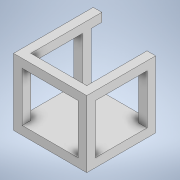
# Autodesk Inventor part: Pump and motor housing new
Saved by Autodesk Inventor 2021 (Build 250183000, 183)
## iProperties
Created: 2020-10-21
Part Number: Pump and motor housing new
Material: Generic
Document SubType Name: Modeling
Designer: nabee
Density: 1 g/cm^3
Appearance: Default
Author: nabee
Autodesk Inventor part; units mm, degrees
ref_plane "YZ Plane" through (0, 0, 0) normal (1, 0, 0) x (0, 1, 0)
ref_plane "XZ Plane" through (0, 0, 0) normal (0, 1, 0) x (-1, 0, 0)
ref_plane "XY Plane" through (0, 0, 0) normal (0, 0, 1) x (1, 0, 0)
sketch "Sketch1" plane through (0, 0, 0) normal (0, 0, 1) x (1, 0, 0)
  line L0 (0, 0) -> (170, 0)
  line L1 (170, 0) -> (170, 310)
  line L2 (170, 310) -> (0, 310)
  line L3 (0, 310) -> (0, 0)
  dimension "d0" = 310
  dimension "d1" = 170
  constraints: 8 end point, 2 parallel, 1 horizontal, 1 perpendicular
  measures "d0" distance of L2.end L0.start
  measures "d1" distance of L0.start L0.end
extrude "Extrusion1" add sketch "Sketch1" along normal blind 150
sketch "Sketch2" plane through (0, 0, 150) normal (0, 0, 1) x (1, 0, 0)
  line L0 (20, 290) -> (150, 290)
  line L1 (150, 290) -> (150, 20)
  line L2 (150, 20) -> (20, 20)
  line L3 (20, 20) -> (20, 290)
  line L4 (170, 310) -> (0, 310) projected
  line L5 (0, 310) -> (0, 0) projected
  line L6 (0, 0) -> (170, 0) projected
  line L7 (170, 0) -> (170, 310) projected
  dimension "d4" = 20
  dimension "d5" = 20
  dimension "d6" = 20
  dimension "d7" = 20
  constraints: 8 end point, 2 parallel, 1 horizontal, 1 perpendicular
  measures "d4" distance between parallel lines of L4 L0
  measures "d5" distance between parallel lines of L5 L3
  measures "d6" distance between parallel lines of L6 L2
  measures "d7" distance between parallel lines of L7 L1
sketch "Sketch3" plane through (0, 310, 0) normal (0, 1, 0) x (1, 0, 0)
  line L0 (20, -20) -> (150, -20)
  line L1 (150, -20) -> (150, -130)
  line L2 (150, -130) -> (20, -130)
  line L3 (20, -130) -> (20, -20)
  line L4 (170, 0) -> (0, 0) projected
  line L5 (0, 0) -> (0, -150) projected
  line L6 (170, -150) -> (0, -150) projected
  line L7 (170, 0) -> (170, -150) projected
  dimension "d8" = 20
  dimension "d9" = 20
  dimension "d10" = 20
  dimension "d11" = 20
  constraints: 8 end point, 2 parallel, 1 horizontal, 1 perpendicular
  measures "d8" distance between parallel lines of L4 L0
  measures "d9" distance between parallel lines of L5 L3
  measures "d10" distance between parallel lines of L6 L2
  measures "d11" distance between parallel lines of L7 L1
sketch "Sketch4" plane through (170, 0, 0) normal (1, 0, 0) x (0, 0, -1)
  line L0 (-130, 290) -> (-20, 290)
  line L1 (-20, 290) -> (-20, 20)
  line L2 (-20, 20) -> (-130, 20)
  line L3 (-130, 20) -> (-130, 290)
  line L4 (0, 310) -> (-150, 310) projected
  line L5 (-150, 0) -> (-150, 310) projected
  line L6 (0, 0) -> (-150, 0) projected
  line L7 (0, 0) -> (0, 310) projected
  dimension "d12" = 20
  dimension "d13" = 20
  dimension "d14" = 20
  dimension "d15" = 20
  constraints: 8 end point, 2 parallel, 1 horizontal, 1 perpendicular
  measures "d12" distance between parallel lines of L4 L0
  measures "d13" distance between parallel lines of L5 L3
  measures "d14" distance between parallel lines of L6 L2
  measures "d15" distance between parallel lines of L7 L1
extrude "Extrusion2" cut sketch "Sketch4" against normal blind 900 contours L0 L1 L2 L3
extrude "Extrusion3" cut sketch "Sketch2" against normal blind 900 contours L0 L1 L2 L3
extrude "Extrusion4" cut sketch "Sketch3" against normal blind 40 contours L0 L1 L2 L3
sketch "Sketch5" plane through (170, 0, 0) normal (1, 0, 0) x (0, 0, -1)
  line L0 (-150, 0) -> (-150, 310) projected
  line L1 (-150, 310) -> (0, 310)
  line L2 (0, 310) -> (0, 135)
  line L3 (0, 135) -> (-150, 135)
  line L4 (-150, 135) -> (-150, 310)
  point P0 (0, 0)
  point P1 (-150, 135)
  dimension "d22" = 175
  constraints: 8 end point, 2 parallel, 1 horizontal, 1 perpendicular
  measures "d22" distance of L1.end L2.end
extrude "Extrusion5" cut sketch "Sketch5" against normal through all
sketch "Sketch6" plane through (0, 0, 150) normal (0, 0, 1) x (1, 0, 0)
  line L0 (20, 135) -> (0, 135) projected
  line L1 (0, 135) -> (20, 135)
  line L2 (20, 135) -> (20, 20)
  line L3 (0, 20) -> (0, 135)
  line L4 (0, 0) -> (170, 0) projected
  line L5 (0, 0) -> (170, 0)
  line L6 (170, 0) -> (170, 20)
  line L7 (0, 20) -> (0, 0)
  line L8 (150, 135) -> (170, 135)
  line L9 (170, 135) -> (170, 20)
  line L10 (150, 20) -> (150, 135)
  line L11 (20, 20) -> (150, 20) projected
  line L12 (20, 20) -> (150, 20)
  constraints: 20 end point, 4 equal length, 3 horizontal, 3 perpendicular
extrude "Extrusion6" add sketch "Sketch6" along normal blind 10
sketch "Sketch7" plane through (170, 20, 130) normal (1, 0, 0) x (0, 0, -1)
  line L0 (0, 115) -> (-30, 115) projected
  line L1 (-30, 0) -> (0, 0) projected
  line L2 (0, 115) -> (-10, 115)
  line L3 (-10, 115) -> (-10, 0)
  line L4 (-10, 0) -> (0, 0)
  line L5 (0, 0) -> (0, 115)
  point P0 (130, -20)
  point P1 (-10, 115)
  dimension "d27" = 10
  constraints: 8 end point, 2 parallel, 1 horizontal, 1 perpendicular, 1 point on line
  measures "d27" distance of L4.end L3.end
extrude "Extrusion7" cut sketch "Sketch7" against normal through all
sketch "Sketch8" plane through (0, 20, 20) normal (0, 0, 1) x (1, 0, 0)
  line L0 (20, 115) -> (20, 0) projected
  line L1 (0, 115) -> (20, 115)
  line L2 (20, 115) -> (20, 95)
  line L3 (20, 95) -> (0, 95)
  line L4 (0, 95) -> (0, 115)
  point P0 (0, -20)
  dimension "d30" = 20
  constraints: 8 end point, 2 parallel, 1 horizontal, 1 perpendicular, 1 point on line
  measures "d30" distance of L3.end L1.start
sketch "Sketch9" plane through (150, 20, 20) normal (0, 0, 1) x (1, 0, 0)
  line L0 (20, 115) -> (20, 0) projected
  line L1 (20, 115) -> (0, 115)
  line L2 (0, 115) -> (0, 95)
  line L3 (0, 95) -> (20, 95)
  line L4 (20, 95) -> (20, 115)
  point P0 (-150, -20)
  point P1 (20, 95)
  dimension "d31" = 20
  constraints: 8 end point, 2 parallel, 1 horizontal, 1 perpendicular
  measures "d31" distance of L1.end L2.end
extrude "Extrusion8" add sketch "Sketch8" along normal up to surface (120 mm away)
extrude "Extrusion9" add sketch "Sketch9" along normal up to surface (120 mm away)
sketch "Sketch10" plane through (0, 135, 0) normal (0, 1, 0) x (1, 0, 0)
  line L0 (0, -160) -> (0, 0) projected
  line L1 (20, 0) -> (20, -160) projected
  line L2 (0, 0) -> (20, 0)
  line L3 (20, 0) -> (20, -160)
  line L4 (20, -160) -> (0, -160)
  line L5 (0, -160) -> (0, 0)
  line L6 (0, 0) -> (170, 0) projected
  line L7 (150, -140) -> (150, -160) projected
  line L8 (170, 0) -> (150, 0)
  line L9 (150, 0) -> (150, -160)
  line L10 (150, -160) -> (170, -160)
  line L11 (170, -160) -> (170, 0)
  point P0 (150, 0)
  constraints: 16 end point, 4 parallel, 2 horizontal, 2 perpendicular
extrude "Extrusion10" add sketch "Sketch10" along normal blind 10
sketch "Sketch11" plane through (170, 0, 160) normal (1, 0, 0) x (0, 0, -1)
  line L0 (140, 115) -> (20, 115) projected
  line L1 (20, 115) -> (140, 115)
  line L2 (140, 115) -> (140, 125)
  line L3 (140, 125) -> (20, 125)
  line L4 (20, 125) -> (20, 115)
  point P0 (160, 0)
  dimension "d38" = 10
  constraints: 8 end point, 2 parallel, 1 horizontal, 1 perpendicular
  measures "d38" distance of L3.end L0.end
extrude "Extrusion11" cut sketch "Sketch11" against normal through all
sketch "Sketch12" plane through (0, 145, 0) normal (0, 1, 0) x (1, 0, 0)
  line L0 (20, -160) -> (20, -140) projected
  line L1 (0, 0) -> (20, 0)
  line L2 (20, 0) -> (20, -160)
  line L3 (20, -160) -> (0, -160)
  line L4 (0, -160) -> (0, 0)
  line L5 (170, 0) -> (170, -160) projected
  line L6 (170, 0) -> (150, 0)
  line L7 (150, 0) -> (150, -160)
  line L8 (150, -160) -> (170, -160)
  line L9 (170, -160) -> (170, 0)
  constraints: 16 end point, 4 parallel, 2 horizontal, 2 perpendicular
extrude "Extrusion12" add sketch "Sketch12" along normal blind 5
sketch "Sketch13" plane through (170, 0, 160) normal (1, 0, 0) x (0, 0, -1)
  line L0 (20, 125) -> (140, 125) projected
  line L1 (20, 125) -> (140, 125)
  line L2 (140, 125) -> (140, 130)
  line L3 (140, 130) -> (20, 130)
  line L4 (20, 130) -> (20, 125)
  point P0 (160, 0)
  dimension "d43" = 5
  constraints: 8 end point, 2 parallel, 1 horizontal, 1 perpendicular
  measures "d43" distance of L3.end L0.start
extrude "Extrusion13" cut sketch "Sketch13" against normal through all
sketch "Sketch14" plane through (0, 150, 0) normal (0, 1, 0) x (1, 0, 0)
  line L0 (20, -160) -> (20, -140) projected
  line L1 (0, 0) -> (20, 0)
  line L2 (20, 0) -> (20, -160)
  line L3 (20, -160) -> (0, -160)
  line L4 (0, -160) -> (0, 0)
  line L5 (0, 0) -> (170, 0) projected
  line L6 (150, -160) -> (20, -160) projected
  line L7 (170, 0) -> (150, 0)
  line L8 (150, 0) -> (150, -160)
  line L9 (150, -160) -> (170, -160)
  line L10 (170, -160) -> (170, 0)
  constraints: 16 end point, 4 parallel, 2 horizontal, 2 perpendicular
extrude "Extrusion14" add sketch "Sketch14" along normal blind 5 contours L3 L4 L1 L2 L0 | L8 L5 L10 L9
sketch "Sketch15" plane through (170, 0, 160) normal (1, 0, 0) x (0, 0, -1)
  line L0 (20, 130) -> (140, 130) projected
  line L1 (20, 130) -> (140, 130)
  line L2 (140, 130) -> (140, 135)
  line L3 (140, 135) -> (20, 135)
  line L4 (20, 135) -> (20, 130)
  point P0 (160, 0)
  dimension "d48" = 5
  constraints: 8 end point, 2 parallel, 1 horizontal, 1 perpendicular
  measures "d48" distance of L3.end L0.start
extrude "Extrusion15" cut sketch "Sketch15" against normal through all
sketch "Sketch17" plane through (0, 0, 0) normal (0, 0, -1) x (-1, 0, 0)
  line L0 (0, 155) -> (-20, 155) projected
  line L1 (0, 155) -> (-20, 155)
  line L2 (-20, 155) -> (-20, 135)
  line L3 (-20, 135) -> (0, 135)
  line L4 (0, 135) -> (0, 155)
  point P0 (0, 0)
  dimension "d52" = 20
  constraints: 8 end point, 2 parallel, 1 horizontal, 1 perpendicular
  measures "d52" distance of L3.end L0.start
extrude "Extrusion16" add sketch "Sketch17" along normal blind 25.003
sketch "Sketch18" plane through (20, 20, 20) normal (1, 0, 0) x (0, 0, -1)
  line L0 (-140, 135) -> (20, 135) projected
  line L1 (-120, 115) -> (0, 115) projected
  line L2 (-140, 135) -> (-120, 135)
  line L3 (-120, 135) -> (-120, 115)
  line L4 (-120, 115) -> (-140, 115)
  line L5 (-140, 115) -> (-140, 135)
  point P0 (20, -20)
  point P1 (-120, 135)
  constraints: 8 end point, 2 parallel, 1 horizontal, 1 perpendicular
extrude "Extrusion17" add sketch "Sketch18" along normal up to surface (130 mm away)
body "Solid1"
